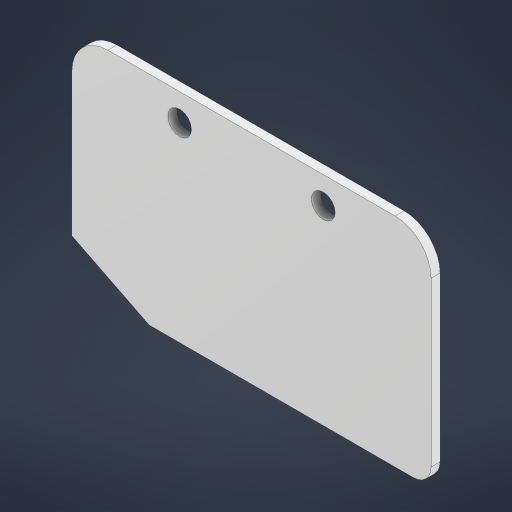
# Autodesk Inventor part: wedge
Saved by Autodesk Inventor 2024 (Build 280153000, 153)
## iProperties
Created: 2023-11-21
Part Number: wedge
Material: Acetal Resin, White
Document SubType Name: Sheet Metal
Designer: avere
Density: 1.425 g/cm^3
Appearance: Smooth - White
Flat Pattern Width: 3.84261 cm
Flat Pattern Length: 6.35 cm
Flat Pattern Area: 24.4006 cm^2
Sheet Metal Rule: Default
Sheet Metal Width: 1.513 in
Sheet Metal Length: 2.500 in
Sheet Metal Area: 3.782 in^2
Author: avere
Autodesk Inventor part; units mm, degrees
ref_plane "YZ Plane" through (0, 0, 0) normal (1, 0, 0) x (0, 1, 0)
ref_plane "XZ Plane" through (0, 0, 0) normal (0, 1, 0) x (-1, 0, 0)
ref_plane "XY Plane" through (0, 0, 0) normal (0, 0, 1) x (1, 0, 0)
sketch "Sketch1" plane through (0, 0, 0) normal (0, 0, 1) x (1, 0, 0)
  circle A0 centre (0, 0) radius 2.0955
  circle A1 centre (25.4, 0) radius 2.0955
  line L0 (-5.3932, -33.6636) -> (41.275, -33.6636)
  line L1 (-12.7, 4.7625) -> (38.1, 4.7625)
  line L2 (-15.875, -9.525) -> (44.45, -9.525)
  line L3 (-19.05, -1.5875) -> (-19.05, -26.8352)
  line L4 (-19.05, -26.8352) -> (-5.3932, -33.6636)
  line L5 (44.45, -1.5875) -> (44.45, -30.4886)
  line L6 (-19.05, -9.525) -> (-15.875, -9.525)
  arc A2 (-12.7, 4.7625) -> (-19.05, -1.5875) centre (-12.7, -1.5875) ccw
  arc A3 (44.45, -1.5875) -> (38.1, 4.7625) centre (38.1, -1.5875) ccw
  arc A4 (41.275, -33.6636) -> (44.45, -30.4886) centre (41.275, -30.4886) ccw
  point P0 (25.4, 4.7625)
  point P1 (28.575, -33.6636)
  point P2 (-19.05, 4.7625)
  point P3 (44.45, 4.7625)
  point P4 (44.45, -30.1625)
  dimension "d0" = 4.191
  dimension "d10" = 6.35
  dimension "d11" = 3.175
  constraints: 14 end point, 9 point on line, 6 point on circle, 6 tangent, 5 centre point, 4 vertical, 1 coincident, 1 collinear, 1 equal radius, 1 horizontal, 2 other
  measures "d0" diameter of A0
  measures "d10" radius of A2
  measures "d11" radius of A4
extrude "Extrusion1" add sketch "Sketch1" along normal blind 1.5875
feature "Bend Part1" [suppressed]
equation "\"BendRadius\" = Thickness"
equation "\"BendReliefWidth\" = Thickness"
equation "\"BendReliefDepth\" = 0.5 * Thickness"
equation "\"CornerReliefSize\" = 4 * Thickness"
equation "\"MinimumRemnant\" = 2 * Thickness"
equation "\"TransitionRadius\" = BendRadius"
equation "\"JacobiRadiusSize\" = BendRadius"
equation "\"GapSize\" = Thickness"
equation "\"Thickness\" = 1.5875"
body "Solid1"
